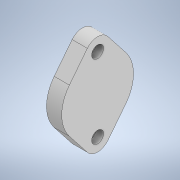
# Autodesk Inventor part: Сборка 13В крышка
Saved by Autodesk Inventor 2021 (Build 250183000, 183)
## iProperties
Created: 2021-03-24
Part Number: Сборка 13В крышка
Material: Типовые
Document SubType Name: Modeling
Designer: khosta
Density: 1 g/cm^3
Appearance: По умолчанию
Author: khosta
Autodesk Inventor part; units mm, degrees
ref_plane "YZ Plane" through (0, 0, 0) normal (1, 0, 0) x (0, 1, 0)
ref_plane "XZ Plane" through (0, 0, 0) normal (0, 1, 0) x (-1, 0, 0)
ref_plane "XY Plane" through (0, 0, 0) normal (0, 0, 1) x (1, 0, 0)
sketch "Эскиз1" plane through (0, 0, 0) normal (1, 0, 0) x (0, 1, 0)
  arc A0 (41.4118, -9.4375) -> (41.4118, 9.4375) centre (34, 0) ccw
  line L0 (41.4118, -9.4375) -> (20.3824, -25.953)
  line L1 (41.4118, 9.4375) -> (20.3824, 25.953)
  arc A1 (20.3824, 25.953) -> (0, 33) centre (0, 0) ccw
  arc A2 (0, -33) -> (20.3824, -25.953) centre (0, 0) ccw
  arc A3 (-41.4118, 9.4375) -> (-41.4118, -9.4375) centre (-34, 0) ccw
  line L2 (-41.4118, -9.4375) -> (-20.3824, -25.953)
  line L3 (-41.4118, 9.4375) -> (-20.3824, 25.953)
  arc A4 (0, 33) -> (-20.3824, 25.953) centre (0, 0) ccw
  arc A5 (-20.3824, -25.953) -> (0, -33) centre (0, 0) ccw
  constraints: 12 point on circle, 8 end point, 6 centre point, 2 tangent
extrude "Выдавливание1" add sketch "Эскиз1" along normal blind 14
sketch "Эскиз2" plane through (0, 0, 0) normal (-1, 0, 0) x (0, 0, 1)
  arc A0 (9.4375, 41.4118) -> (-9.4375, 41.4118) centre (0, 34) ccw projected
  point P0 (0, 0)
  point P1 (0, -34)
  constraints: 1 coincident
hole "Отверстие1" at (0, -34, 0) at (0, 34, 0) direction (1, 0, 0) diameter 11 end through all counterbore diameter 18 counterbore depth 7
